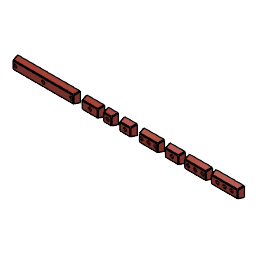
Keycaps Print (Autodesk Fusion 360 design; units mm, degrees)
part number: 2026-04-15-17-36-02-088
Autodesk Fusion 360 part; units mm, degrees
(part 1 of 2)
sketch "Sketch1" plane through (0, 0, 0) normal (0, 1, 0) x (1, 0, 0)
  line L0 (0, 0) -> (18, 0)
  line L1 (18, 0) -> (18, 18)
  line L2 (18, 18) -> (0, 18)
  line L3 (0, 18) -> (0, 0)
  dimension "d1" = 18
  dimension "d2" = 18
  constraint horizontal L0
  constraint vertical L1
  constraint horizontal L2
  constraint vertical L3
  constraint coincident L0.start L3.end
  measures "d1" distance of L0.start L0.end
  measures "d2" distance of L0.start L2.end
extrude "Extrude1" add sketch "Sketch1" along normal blind 10 makes body 1
sketch "Sketch2" plane through (0, 0, 0) normal (0, 0, 1) x (1, 0, 0)
  line L0 (0, 0) -> (18, 0)
  line L1 (18, 0) -> (18, 10)
  line L2 (18, 10) -> (0, 10)
  line L3 (0, 10) -> (0, 0)
  line L4 (0, 10) -> (2, 10)
  line L5 (2, 10) -> (0, 0)
  line L6 (0, 0) -> (0, 10)
  line L7 (18, 10) -> (16, 10)
  line L8 (16, 10) -> (18, 0)
  line L9 (18, 0) -> (18, 10)
  constraint coincident L2.end L3.start
  constraint coincident L2 L4.end
  constraint coincident L0.start L3.end
  constraint coincident L1.end L2.start
  constraint coincident L2 L7.end
  constraint coincident L0.end L1.start
sketch "Sketch3" plane through (18, 0, 0) normal (1, 0, 0) x (0, 0, -1)
  line L0 (0, 0) -> (18, 0)
  line L1 (18, 0) -> (18, 10)
  line L2 (18, 10) -> (0, 10)
  line L3 (0, 10) -> (0, 0)
  line L4 (0, 10) -> (2, 10)
  line L5 (2, 10) -> (0, 0)
  line L6 (0, 0) -> (0, 10)
  line L7 (18, 10) -> (16, 10)
  line L8 (16, 10) -> (18, 0)
  line L9 (18, 0) -> (18, 10)
  constraint coincident L2.end L3.start
  constraint coincident L2 L4.end
  constraint coincident L0.start L3.end
  constraint coincident L1.end L2.start
  constraint coincident L2 L7.end
  constraint coincident L0.end L1.start
extrude "Extrude2" cut sketch "Sketch3" against normal blind 39 contours L2 L3 L4 L5 L6 | L1 L2 L7 L8 L9 bodies 1
extrude "Extrude3" cut sketch "Sketch2" against normal blind 27 contours L2 L3 L4 L5 L6 | L1 L2 L7 L8 L9 bodies 1
shell "Shell2" thickness 1 removed faces 1 at (6, 0, -12) on bodies 1
sketch "Sketch4" plane through (0, 9, 0) normal (0, -1, 0) x (1, 0, 0)
  line L0 (15.1802, -15.1802) -> (15.1802, -2.8198)
  line L1 (15.1802, -2.8198) -> (2.8198, -2.8198)
  line L2 (2.8198, -2.8198) -> (2.8198, -15.1802)
  line L3 (2.8198, -15.1802) -> (15.1802, -15.1802)
  line L4 (8.45, -11) -> (9.55, -11)
  line L5 (9.55, -11) -> (9.55, -7)
  line L6 (9.55, -7) -> (8.45, -7)
  line L7 (8.45, -7) -> (8.45, -11)
  line L8 (7, -8.375) -> (11, -8.375)
  line L9 (11, -8.375) -> (11, -9.625)
  line L10 (11, -9.625) -> (7, -9.625)
  line L11 (7, -9.625) -> (7, -8.375)
  line L12 (10.55, -6) -> (7.45, -6)
  line L13 (7.45, -6) -> (7.45, -12)
  line L14 (7.45, -12) -> (10.55, -12)
  line L15 (10.55, -12) -> (10.55, -6)
  line L16 (12, -10.625) -> (6, -10.625)
  line L17 (6, -10.625) -> (6, -7.375)
  line L18 (6, -7.375) -> (12, -7.375)
  line L19 (12, -7.375) -> (12, -10.625)
  dimension "d21" = 3.1
  dimension "d22" = 6
  dimension "d25" = 6
  dimension "d26" = 3.25
  constraint horizontal L4
  constraint vertical L5
  constraint horizontal L6
  constraint vertical L7
  constraint horizontal L8
  constraint vertical L9
  constraint horizontal L10
  constraint vertical L11
  constraint horizontal L12
  constraint vertical L13
  constraint horizontal L14
  constraint vertical L15
  constraint horizontal L16
  constraint vertical L17
  constraint horizontal L18
  constraint vertical L19
  measures "d21" distance of L12.start L12.end
  measures "d22" distance of L12.start L14.end
  measures "d25" distance of L16.start L16.end
  measures "d26" distance of L16.start L18.end
extrude "Extrude4" add sketch "Sketch4" along normal blind 9 contours L4 L5 L7 L13 L14 L15 L16 | L7 L10 L13 L16 | L5 L10 L15 L16 | L8 L10 L11 L13 L16 L17 L18 | L8 L9 L10 L15 L16 L18 L19 | L7 L8 L13 L18 | L5 L8 L15 L18 | L5 L6 L7 L12 L13 L15 L18 bodies 1
fillet "Fillet1" radius 1 8 edges at (16, 10, -9) (9, 10, -16) (2, 10, -9) (9, 10, -2) (1, 5, -17) (1, 5, -1) (17, 5, -1) (17, 5, -17) on bodies 1
move_body "Move1" bodies 1 to x (1, 0, 0) y (0, 0, 1) z (0, -1, 0) at (-9, -1.3198, -24.8198)
move_body "Move2" bodies 1 to x (1, 0, 0) y (0, 1, 0) z (0, 0, 1) at (0, -7, 37)
sketch "Sketch5" plane through (0, 0, 0) normal (0, 0, 1) x (1, 0, 0)
  line L0 (25, 0) -> (133, 0)
  line L1 (133, 0) -> (133, 18)
  line L2 (133, 18) -> (25, 18)
  line L3 (25, 18) -> (25, 0)
  dimension "d31" = 108
  dimension "d32" = 18
  constraint horizontal L0
  constraint vertical L1
  constraint horizontal L2
  constraint vertical L3
  measures "d31" distance of L0.start L0.end
  measures "d32" distance of L0.start L2.end
extrude "Extrude5" add sketch "Sketch5" along normal blind 10 separate body makes body 2
sketch "Sketch6" plane through (0, 0, 0) normal (0, -1, 0) x (1, 0, 0)
  line L0 (25, 0) -> (133, 0)
  line L1 (133, 0) -> (133, 10)
  line L2 (133, 10) -> (25, 10)
  line L3 (25, 10) -> (25, 0)
  line L4 (25, 10) -> (27, 10)
  line L5 (27, 10) -> (25, 0)
  line L6 (25, 0) -> (25, 10)
  line L7 (133, 10) -> (131, 10)
  line L8 (131, 10) -> (133, 0)
  line L9 (133, 0) -> (133, 10)
  constraint coincident L2.end L3.start
  constraint coincident L2 L4.end
  constraint coincident L0.start L3.end
  constraint coincident L1.end L2.start
  constraint coincident L2 L7.end
  constraint coincident L0.end L1.start
sketch "Sketch7" plane through (133, 0, 0) normal (1, 0, 0) x (0, 0, -1)
  line L0 (0, 0) -> (0, 18)
  line L1 (0, 18) -> (-10, 18)
  line L2 (-10, 18) -> (-10, 0)
  line L3 (-10, 0) -> (0, 0)
  line L4 (-10, 0) -> (-10, 2)
  line L5 (-10, 2) -> (0, 0)
  line L6 (0, 0) -> (-10, 0)
  line L7 (-10, 18) -> (-10, 16)
  line L8 (-10, 16) -> (0, 18)
  line L9 (0, 18) -> (-10, 18)
  constraint coincident L2.end L3.start
  constraint coincident L2 L4.end
  constraint coincident L0.start L3.end
  constraint coincident L1.end L2.start
  constraint coincident L2 L7.end
  constraint coincident L0.end L1.start
extrude "Extrude6" cut sketch "Sketch7" against normal blind 116 contours L2 L3 L4 L5 L6 | L1 L2 L7 L8 L9 bodies 2
extrude "Extrude7" cut sketch "Sketch6" against normal blind 20 contours L2 L3 L4 L5 L6 | L1 L2 L7 L8 L9 bodies 2
shell "Shell3" thickness 1 removed faces 1 at (61, 12, 0) on bodies 2
sketch "Sketch8" plane through (0, 0, 9) normal (0, 0, -1) x (-1, 0, 0)
  line L0 (-27.8198, 2.8198) -> (-27.8198, 15.1802)
  line L1 (-27.8198, 15.1802) -> (-130.1802, 15.1802)
  line L2 (-130.1802, 15.1802) -> (-130.1802, 2.8198)
  line L3 (-130.1802, 2.8198) -> (-27.8198, 2.8198)
  line L4 (-79.55, 7) -> (-78.45, 7)
  line L5 (-78.45, 7) -> (-78.45, 11)
  line L6 (-78.45, 11) -> (-79.55, 11)
  line L7 (-79.55, 11) -> (-79.55, 7)
  line L8 (-77, 8.375) -> (-81, 8.375)
  line L9 (-81, 8.375) -> (-81, 9.625)
  line L10 (-81, 9.625) -> (-77, 9.625)
  line L11 (-77, 9.625) -> (-77, 8.375)
  line L12 (-80.55, 6) -> (-77.45, 6)
  line L13 (-77.45, 6) -> (-77.45, 12)
  line L14 (-77.45, 12) -> (-80.55, 12)
  line L15 (-80.55, 12) -> (-80.55, 6)
  line L16 (-82, 7.375) -> (-76, 7.375)
  line L17 (-76, 7.375) -> (-76, 10.625)
  line L18 (-76, 10.625) -> (-82, 10.625)
  line L19 (-82, 10.625) -> (-82, 7.375)
  line L20 (-123.788, 10.625) -> (-129.788, 10.625)
  line L21 (-129.788, 10.625) -> (-129.788, 7.375)
  line L22 (-129.788, 7.375) -> (-123.788, 7.375)
  line L23 (-123.788, 7.375) -> (-123.788, 10.625)
  line L24 (-128.788, 9.625) -> (-124.788, 9.625)
  line L25 (-124.788, 9.625) -> (-124.788, 8.375)
  line L26 (-128.788, 8.375) -> (-128.788, 9.625)
  line L27 (-124.788, 8.375) -> (-128.788, 8.375)
  line L28 (-127.338, 11) -> (-127.338, 7)
  line L29 (-127.338, 7) -> (-126.238, 7)
  line L30 (-126.238, 11) -> (-127.338, 11)
  line L31 (-126.238, 7) -> (-126.238, 11)
  line L32 (-128.338, 12) -> (-128.338, 6)
  line L33 (-128.338, 6) -> (-125.238, 6)
  line L34 (-125.238, 12) -> (-128.338, 12)
  line L35 (-125.238, 6) -> (-125.238, 12)
  line L36 (-76, 10.625) -> (-82, 10.625)
  line L37 (-82, 10.625) -> (-82, 7.375)
  line L38 (-82, 7.375) -> (-76, 7.375)
  line L39 (-76, 7.375) -> (-76, 10.625)
  line L40 (-81, 9.625) -> (-77, 9.625)
  line L41 (-77, 9.625) -> (-77, 8.375)
  line L42 (-81, 8.375) -> (-81, 9.625)
  line L43 (-77, 8.375) -> (-81, 8.375)
  line L44 (-79.55, 11) -> (-79.55, 7)
  line L45 (-79.55, 7) -> (-78.45, 7)
  line L46 (-78.45, 11) -> (-79.55, 11)
  line L47 (-78.45, 7) -> (-78.45, 11)
  line L48 (-80.55, 12) -> (-80.55, 6)
  line L49 (-80.55, 6) -> (-77.45, 6)
  line L50 (-77.45, 12) -> (-80.55, 12)
  line L51 (-77.45, 6) -> (-77.45, 12)
  line L52 (-28.212, 10.625) -> (-34.212, 10.625)
  line L53 (-34.212, 10.625) -> (-34.212, 7.375)
  line L54 (-34.212, 7.375) -> (-28.212, 7.375)
  line L55 (-28.212, 7.375) -> (-28.212, 10.625)
  line L56 (-33.212, 9.625) -> (-29.212, 9.625)
  line L57 (-29.212, 9.625) -> (-29.212, 8.375)
  line L58 (-33.212, 8.375) -> (-33.212, 9.625)
  line L59 (-29.212, 8.375) -> (-33.212, 8.375)
  line L60 (-31.762, 11) -> (-31.762, 7)
  line L61 (-31.762, 7) -> (-30.662, 7)
  line L62 (-30.662, 11) -> (-31.762, 11)
  line L63 (-30.662, 7) -> (-30.662, 11)
  line L64 (-32.762, 12) -> (-32.762, 6)
  line L65 (-32.762, 6) -> (-29.662, 6)
  line L66 (-29.662, 12) -> (-32.762, 12)
  line L67 (-29.662, 6) -> (-29.662, 12)
  dimension "d46" = 3.1
  dimension "d47" = 6
  dimension "d50" = 6
  dimension "d51" = 3.25
  dimension "d56" = 3.1
  dimension "d57" = 6
  dimension "d58" = 6
  dimension "d59" = 3.25
  dimension "d60" = 3.1
  dimension "d61" = 6
  dimension "d62" = 6
  dimension "d63" = 3.25
  dimension "d64" = 3.1
  dimension "d65" = 6
  dimension "d66" = 6
  dimension "d67" = 3.25
  constraint horizontal L4
  constraint vertical L5
  constraint horizontal L6
  constraint vertical L7
  constraint horizontal L8
  constraint vertical L9
  constraint horizontal L10
  constraint vertical L11
  constraint horizontal L12
  constraint vertical L13
  constraint horizontal L14
  constraint vertical L15
  constraint horizontal L16
  constraint vertical L17
  constraint horizontal L18
  constraint vertical L19
  constraint horizontal L29
  constraint vertical L31
  constraint horizontal L30
  constraint vertical L28
  constraint horizontal L27
  constraint vertical L26
  constraint horizontal L24
  constraint vertical L25
  constraint horizontal L33
  constraint vertical L35
  constraint horizontal L34
  constraint vertical L32
  constraint horizontal L22
  constraint vertical L23
  constraint horizontal L20
  constraint vertical L21
  constraint horizontal L45
  constraint vertical L47
  constraint horizontal L46
  constraint vertical L44
  constraint horizontal L43
  constraint vertical L42
  constraint horizontal L40
  constraint vertical L41
  constraint horizontal L49
  constraint vertical L51
  constraint horizontal L50
  constraint vertical L48
  constraint horizontal L38
  constraint vertical L39
  constraint horizontal L36
  constraint vertical L37
  constraint horizontal L61
  constraint vertical L63
  constraint horizontal L62
  constraint vertical L60
  constraint horizontal L59
  constraint vertical L58
  constraint horizontal L56
  constraint vertical L57
  constraint horizontal L65
  constraint vertical L67
  constraint horizontal L66
  constraint vertical L64
  constraint horizontal L54
  constraint vertical L55
  constraint horizontal L52
  constraint vertical L53
  measures "d46" distance of L12.start L12.end
  measures "d47" distance of L12.start L14.end
  measures "d50" distance of L16.start L16.end
  measures "d51" distance of L16.start L18.end
  measures "d56" distance of L33.end L32.end
  measures "d57" distance of L32.start L32.end
  measures "d58" distance of L22.end L21.end
  measures "d59" distance of L20.end L21.end
  measures "d60" distance of L12.end L12.start
  measures "d61" distance of L14.end L12.start
  measures "d62" distance of L16.end L16.start
  measures "d63" distance of L18.end L16.start
  measures "d64" distance of L65.end L64.end
  measures "d65" distance of L64.start L64.end
  measures "d66" distance of L54.end L53.end
  measures "d67" distance of L52.end L53.end
extrude "Extrude8" add sketch "Sketch8" along normal blind 9 contours L4 L5 L7 L12 L13 L15 L16 L38 L44 L45 L47 L48 L49 L51 | L7 L8 L15 L16 L38 L43 L44 L48 | L5 L8 L13 L16 L38 L43 L47 L51 | L8 L9 L10 L15 L16 L18 L19 L36 L37 L38 L40 L42 L43 L48 | L8 L10 L11 L13 L16 L17 L18 L36 L38 L39 L40 L41 L43 L51 | L7 L10 L15 L18 L36 L40 L44 L48 | L5 L10 L13 L18 L36 L40 L47 L51 | L5 L6 L7 L13 L14 L15 L18 L36 L44 L46 L47 L48 L50 L51 bodies 2
fillet "Fillet2" radius 1 8 edges at (79, 16, 10) (27, 9, 10) (26, 17, 5) (26, 1, 5) (79, 2, 10) (132, 17, 5) (131, 9, 10) (132, 1, 5) on bodies 2
extrude "Extrude9" add sketch "Sketch8" along normal blind 9 contours L20 L22 L23 L24 L25 L27 L35 | L20 L24 L31 L35 | L20 L28 L30 L31 L32 L34 L35 | L22 L28 L29 L31 L32 L33 L35 | L22 L27 L31 L35 | L20 L24 L28 L32 | L20 L21 L22 L24 L26 L27 L32 | L22 L27 L28 L32 | L52 L54 L55 L56 L57 L59 L67 | L52 L56 L63 L67 | L52 L60 L62 L63 L64 L66 L67 | L54 L60 L61 L63 L64 L65 L67 | L54 L59 L63 L67 | L52 L56 L60 L64 | L52 L53 L54 L56 L58 L59 L64 | L54 L59 L60 L64 bodies 2
move_body "Move3" bodies 2 to x (1, 0, 0) y (0, 1, 0) z (0, 0, 1) at (-78.996, -8.312, 15)
move_body "Move4" bodies 2 to x (1, 0, 0) y (0, 1, 0) z (0, 0, 1) at (0, 0, -2.8)
sketch "Sketch9" plane through (0, 0, 0) normal (0, 0, 1) x (1, 0, 0)
  line L0 (-75, 0) -> (-97.5, 0)
  line L1 (-97.5, 0) -> (-97.5, -18)
  line L2 (-97.5, -18) -> (-75, -18)
  line L3 (-75, -18) -> (-75, 0)
  dimension "d70" = 22.5
  dimension "d71" = 18
  constraint horizontal L0
  constraint vertical L1
  constraint horizontal L2
  constraint vertical L3
  measures "d70" distance of L0.start L0.end
  measures "d71" distance of L0.start L2.end
extrude "Extrude10" add sketch "Sketch9" along normal blind 10 separate body makes body 3
sketch "Sketch10" plane through (0, 0, 0) normal (0, 1, 0) x (-1, 0, 0)
  line L0 (75, 0) -> (97.5, 0)
  line L1 (97.5, 0) -> (97.5, 10)
  line L2 (97.5, 10) -> (75, 10)
  line L3 (75, 10) -> (75, 0)
  line L4 (75, 10) -> (77, 10)
  line L5 (77, 10) -> (75, 0)
  line L6 (75, 0) -> (75, 10)
  line L7 (97.5, 10) -> (95.5, 10)
  line L8 (95.5, 10) -> (97.5, 0)
  line L9 (97.5, 0) -> (97.5, 10)
  dimension "d74" = 2
  constraint coincident L2.end L3.start
  constraint coincident L2 L4.end
  constraint coincident L0.start L3.end
  constraint coincident L1.end L2.start
  constraint perpendicular L1 L7
  constraint coincident L0.end L1.start
  measures "d74" distance of L1.end L7.end
sketch "Sketch11" plane through (-97.5, 0, 0) normal (-1, 0, 0) x (0, 0, 1)
  line L0 (0, 0) -> (0, -18)
  line L1 (0, -18) -> (10, -18)
  line L2 (10, -18) -> (10, 0)
  line L3 (10, 0) -> (0, 0)
  line L4 (10, 0) -> (10, -2)
  line L5 (10, -2) -> (0, 0)
  line L6 (0, 0) -> (10, 0)
  line L7 (10, -18) -> (10, -16)
  line L8 (10, -16) -> (0, -18)
  line L9 (0, -18) -> (10, -18)
  constraint coincident L2.end L3.start
  constraint coincident L2 L4.end
  constraint coincident L0.start L3.end
  constraint coincident L1.end L2.start
  constraint coincident L2 L7.end
  constraint coincident L0.end L1.start
extrude "Extrude11" cut sketch "Sketch11" against normal blind 27 contours L2 L3 L4 L5 L6 | L1 L2 L7 L8 L9 bodies 3
extrude "Extrude12" cut sketch "Sketch10" against normal blind 26 contours L2 L3 L4 L5 L6 | L1 L2 L7 L8 L9 bodies 3
shell "Shell4" thickness 1 removed faces 1 at (-90, -6, 0) on bodies 3
sketch "Sketch12" plane through (0, 0, 9) normal (0, 0, -1) x (-1, 0, 0)
  line L0 (94.6802, -15.1802) -> (94.6802, -2.8198)
  line L1 (94.6802, -2.8198) -> (77.8198, -2.8198)
  line L2 (77.8198, -2.8198) -> (77.8198, -15.1802)
  line L3 (77.8198, -15.1802) -> (94.6802, -15.1802)
  line L4 (85.7, -11) -> (86.8, -11)
  line L5 (86.8, -11) -> (86.8, -7)
  line L6 (86.8, -7) -> (85.7, -7)
  line L7 (85.7, -7) -> (85.7, -11)
  line L8 (84.25, -8.375) -> (88.25, -8.375)
  line L9 (88.25, -8.375) -> (88.25, -9.625)
  line L10 (88.25, -9.625) -> (84.25, -9.625)
  line L11 (84.25, -9.625) -> (84.25, -8.375)
  line L12 (87.8, -6) -> (84.7, -6)
  line L13 (84.7, -6) -> (84.7, -12)
  line L14 (84.7, -12) -> (87.8, -12)
  line L15 (87.8, -12) -> (87.8, -6)
  line L16 (89.25, -10.625) -> (83.25, -10.625)
  line L17 (83.25, -10.625) -> (83.25, -7.375)
  line L18 (83.25, -7.375) -> (89.25, -7.375)
  line L19 (89.25, -7.375) -> (89.25, -10.625)
  dimension "d90" = 3.1
  dimension "d91" = 6
  dimension "d94" = 6
  dimension "d95" = 3.25
  constraint horizontal L4
  constraint vertical L5
  constraint horizontal L6
  constraint vertical L7
  constraint horizontal L8
  constraint vertical L9
  constraint horizontal L10
  constraint vertical L11
  constraint horizontal L12
  constraint vertical L13
  constraint horizontal L14
  constraint vertical L15
  constraint horizontal L16
  constraint vertical L17
  constraint horizontal L18
  constraint vertical L19
  measures "d90" distance of L12.start L12.end
  measures "d91" distance of L12.start L14.end
  measures "d94" distance of L16.start L16.end
  measures "d95" distance of L16.start L18.end
extrude "Extrude13" add sketch "Sketch12" along normal blind 9 contours L4 L5 L7 L13 L14 L15 L16 | L7 L10 L13 L16 | L5 L10 L15 L16 | L8 L10 L11 L13 L16 L17 L18 | L8 L9 L10 L15 L16 L18 L19 | L7 L8 L13 L18 | L5 L8 L15 L18 | L5 L6 L7 L12 L13 L15 L18 bodies 3
fillet "Fillet3" radius 1 8 edges at (-86.25, -16, 10) (-76, -17, 5) (-77, -9, 10) (-76, -1, 5) (-86.25, -2, 10) (-96.5, -17, 5) (-95.5, -9, 10) (-96.5, -1, 5) on bodies 3
move_body "Move5" bodies 3 to x (1, 0, 0) y (0, 1, 0) z (0, 0, 1) at (86.2551, 9.6865, 12)
move_body "Move6" bodies 3 to x (1, 0, 0) y (0, 1, 0) z (0, 0, 1) at (0, 0, 0.2)
sketch "Sketch13" plane through (0, 0, 0) normal (0, 0, 1) x (1, 0, 0)
  line L0 (20, 0) -> (56, 0)
  line L1 (56, 0) -> (56, 18)
  line L2 (56, 18) -> (20, 18)
  line L3 (20, 18) -> (20, 0)
  dimension "d100" = 36
  dimension "d101" = 18
  constraint horizontal L0
  constraint vertical L1
  constraint horizontal L2
  constraint vertical L3
  measures "d100" distance of L0.start L0.end
  measures "d101" distance of L0.start L2.end
extrude "Extrude14" add sketch "Sketch13" along normal blind 10 separate body makes body 4
sketch "Sketch14" plane through (0, 0, 0) normal (0, -1, 0) x (1, 0, 0)
  line L0 (20, 0) -> (56, 0)
  line L1 (56, 0) -> (56, 10)
  line L2 (56, 10) -> (20, 10)
  line L3 (20, 10) -> (20, 0)
  line L4 (20, 10) -> (22, 10)
  line L5 (22, 10) -> (20, 0)
  line L6 (20, 0) -> (20, 10)
  line L7 (56, 10) -> (54, 10)
  line L8 (54, 10) -> (56, 0)
  line L9 (56, 0) -> (56, 10)
  constraint coincident L2.end L3.start
  constraint coincident L2 L4.end
  constraint coincident L0.start L3.end
  constraint coincident L1.end L2.start
  constraint coincident L2 L7.end
  constraint coincident L0.end L1.start
sketch "Sketch15" plane through (56, 0, 0) normal (1, 0, 0) x (0, 0, -1)
  line L0 (0, 0) -> (0, 18)
  line L1 (0, 18) -> (-10, 18)
  line L2 (-10, 18) -> (-10, 0)
  line L3 (-10, 0) -> (0, 0)
  line L4 (-10, 0) -> (-10, 2)
  line L5 (-10, 2) -> (0, 0)
  line L6 (0, 0) -> (-10, 0)
  line L7 (-10, 18) -> (-10, 16)
  line L8 (-10, 16) -> (0, 18)
  line L9 (0, 18) -> (-10, 18)
  constraint coincident L2.end L3.start
  constraint coincident L2 L4.end
  constraint coincident L0.start L3.end
  constraint coincident L1.end L2.start
  constraint coincident L2 L7.end
  constraint coincident L0.end L1.start
extrude "Extrude15" cut sketch "Sketch15" against normal blind 41 contours L2 L3 L4 L5 L6 | L1 L2 L7 L8 L9 bodies 4
extrude "Extrude16" cut sketch "Sketch14" against normal blind 32 contours L2 L3 L4 L5 L6 | L1 L2 L7 L8 L9 bodies 4
shell "Shell5" thickness 1 removed faces 1 at (32, 12, 0) on bodies 4
sketch "Sketch16" plane through (0, 0, 9) normal (0, 0, -1) x (-1, 0, 0)
  line L0 (-22.8198, 2.8198) -> (-22.8198, 15.1802)
  line L1 (-22.8198, 15.1802) -> (-53.1802, 15.1802)
  line L2 (-53.1802, 15.1802) -> (-53.1802, 2.8198)
  line L3 (-53.1802, 2.8198) -> (-22.8198, 2.8198)
  line L4 (-38.55, 7) -> (-37.45, 7)
  line L5 (-37.45, 7) -> (-37.45, 11)
  line L6 (-37.45, 11) -> (-38.55, 11)
  line L7 (-38.55, 11) -> (-38.55, 7)
  line L8 (-38, 9) -> (-40, 9)
  line L9 (-40, 9) -> (-40, 9.625)
  line L10 (-40, 9.625) -> (-36, 9.625)
  line L11 (-36, 9.625) -> (-36, 8.375)
  line L12 (-36, 8.375) -> (-40, 8.375)
  line L13 (-40, 8.375) -> (-40, 9.625)
  line L14 (-39.55, 6) -> (-36.45, 6)
  line L15 (-36.45, 6) -> (-36.45, 12)
  line L16 (-36.45, 12) -> (-39.55, 12)
  line L17 (-39.55, 12) -> (-39.55, 6)
  line L18 (-35, 7.375) -> (-41, 7.375)
  line L19 (-41, 7.375) -> (-41, 10.625)
  line L20 (-41, 10.625) -> (-35, 10.625)
  line L21 (-35, 10.625) -> (-35, 7.375)
  line L22 (-22.922, 10.625) -> (-22.922, 7.375)
  line L23 (-22.922, 7.375) -> (-28.922, 7.375)
  line L24 (-28.922, 7.375) -> (-28.922, 10.625)
  line L25 (-28.922, 10.625) -> (-22.922, 10.625)
  line L26 (-24.372, 6) -> (-24.372, 12)
  line L27 (-24.372, 12) -> (-27.472, 12)
  line L28 (-27.472, 6) -> (-24.372, 6)
  line L29 (-27.472, 12) -> (-27.472, 6)
  line L30 (-23.922, 9.625) -> (-23.922, 8.375)
  line L31 (-23.922, 8.375) -> (-27.922, 8.375)
  line L32 (-27.922, 8.375) -> (-27.922, 9.625)
  line L33 (-27.922, 9.625) -> (-23.922, 9.625)
  line L34 (-25.372, 7) -> (-25.372, 11)
  line L35 (-25.372, 11) -> (-26.472, 11)
  line L36 (-26.472, 7) -> (-25.372, 7)
  line L37 (-26.472, 11) -> (-26.472, 7)
  line L38 (-47.078, 10.625) -> (-47.078, 7.375)
  line L39 (-47.078, 7.375) -> (-53.078, 7.375)
  line L40 (-53.078, 7.375) -> (-53.078, 10.625)
  line L41 (-53.078, 10.625) -> (-47.078, 10.625)
  line L42 (-48.528, 6) -> (-48.528, 12)
  line L43 (-48.528, 12) -> (-51.628, 12)
  line L44 (-51.628, 6) -> (-48.528, 6)
  line L45 (-51.628, 12) -> (-51.628, 6)
  line L46 (-48.078, 9.625) -> (-48.078, 8.375)
  line L47 (-48.078, 8.375) -> (-52.078, 8.375)
  line L48 (-52.078, 8.375) -> (-52.078, 9.625)
  line L49 (-52.078, 9.625) -> (-48.078, 9.625)
  line L50 (-49.528, 7) -> (-49.528, 11)
  line L51 (-49.528, 11) -> (-50.628, 11)
  line L52 (-50.628, 7) -> (-49.528, 7)
  line L53 (-50.628, 11) -> (-50.628, 7)
  dimension "d112" = 1.1
  dimension "d113" = 4
  dimension "d115" = 2
  dimension "d116" = 0.625
  dimension "d117" = 4
  dimension "d118" = 1.25
  dimension "d121" = 3.1
  dimension "d122" = 6
  dimension "d125" = 6
  dimension "d126" = 3.25
  dimension "d131" = 1.1
  dimension "d132" = 4
  dimension "d133" = 4
  dimension "d134" = 1.25
  dimension "d135" = 3.1
  dimension "d136" = 6
  dimension "d137" = 6
  dimension "d138" = 3.25
  dimension "d139" = 1.1
  dimension "d140" = 4
  dimension "d141" = 4
  dimension "d142" = 1.25
  dimension "d143" = 3.1
  dimension "d144" = 6
  dimension "d145" = 6
  dimension "d146" = 3.25
  constraint horizontal L4
  constraint vertical L5
  constraint horizontal L6
  constraint vertical L7
  constraint perpendicular L5 L8
  constraint perpendicular L8 L9
  constraint horizontal L10
  constraint vertical L11
  constraint horizontal L12
  constraint vertical L13
  constraint horizontal L14
  constraint vertical L15
  constraint horizontal L16
  constraint vertical L17
  constraint horizontal L18
  constraint vertical L19
  constraint horizontal L20
  constraint vertical L21
  constraint horizontal L36
  constraint vertical L34
  constraint horizontal L35
  constraint vertical L37
  constraint horizontal L33
  constraint vertical L30
  constraint horizontal L31
  constraint vertical L32
  constraint horizontal L28
  constraint vertical L26
  constraint horizontal L27
  constraint vertical L29
  constraint horizontal L23
  constraint vertical L24
  constraint horizontal L25
  constraint vertical L22
  constraint horizontal L52
  constraint vertical L50
  constraint horizontal L51
  constraint vertical L53
  constraint horizontal L49
  constraint vertical L46
  constraint horizontal L47
  constraint vertical L48
  constraint horizontal L44
  constraint vertical L42
  constraint horizontal L43
  constraint vertical L45
  constraint horizontal L39
  constraint vertical L40
  constraint horizontal L41
  constraint vertical L38
  measures "d112" distance of L4.start L4.end
  measures "d113" distance of L4.start L6.end
  measures "d115" distance of L8.start L8.end
  measures "d116" distance of L8.end L9.end
  measures "d117" distance of L9.end L10.end
  measures "d118" distance of L9.end L12.end
  measures "d121" distance of L14.start L14.end
  measures "d122" distance of L14.start L16.end
  measures "d125" distance of L18.start L18.end
  measures "d126" distance of L18.start L20.end
  measures "d131" distance of L36.start L34.start
  measures "d132" distance of L36.start L35.end
  measures "d133" distance of L32.end L30.start
  measures "d134" distance of L32.end L31.end
  measures "d135" distance of L28.start L26.start
  measures "d136" distance of L27.end L28.start
  measures "d137" distance of L23.end L22.end
  measures "d138" distance of L22.end L22.start
  measures "d139" distance of L52.start L50.start
  measures "d140" distance of L52.start L51.end
  measures "d141" distance of L48.end L46.start
  measures "d142" distance of L48.end L47.end
  measures "d143" distance of L44.start L42.start
  measures "d144" distance of L43.end L44.start
  measures "d145" distance of L39.end L38.end
  measures "d146" distance of L38.end L38.start
extrude "Extrude17" add sketch "Sketch16" along normal blind 9 contours L4 L5 L7 L14 L15 L17 L18 | L7 L12 L17 L18 | L5 L12 L15 L18 | L9 L10 L12 L13 L17 L18 L19 L20 | L10 L11 L12 L15 L18 L20 L21 | L5 L10 L15 L20 | L7 L10 L17 L20 | L5 L6 L7 L15 L16 L17 L20 bodies 4
extrude "Extrude18" add sketch "Sketch16" along normal blind 9 contours L22 L23 L25 L26 L30 L31 L33 | L25 L26 L33 L34 | L25 L26 L27 L29 L34 L35 L37 | L23 L26 L28 L29 L34 L36 L37 | L23 L26 L31 L34 | L25 L29 L33 L37 | L23 L29 L31 L37 | L23 L24 L25 L29 L31 L32 L33 | L38 L39 L41 L42 L46 L47 L49 | L41 L42 L49 L50 | L41 L42 L43 L45 L50 L51 L53 | L39 L42 L44 L45 L50 L52 L53 | L39 L42 L47 L50 | L41 L45 L49 L53 | L39 L45 L47 L53 | L39 L40 L41 L45 L47 L48 L49 bodies 4
fillet "Fillet5" radius 1 8 edges at (38, 16, 10) (22, 9, 10) (21, 17, 5) (21, 1, 5) (38, 2, 10) (55, 17, 5) (54, 9, 10) (55, 1, 5) on bodies 4
move_body "Move7" bodies 4 to x (1, 0, 0) y (0, 1, 0) z (0, 0, 1) at (-37.9759, -8.2892, 12)
move_body "Move8" bodies 4 to x (1, 0, 0) y (0, 1, 0) z (0, 0, 1) at (-0.0354, -0.0473, 0)
move_body "Move9" bodies 4 to x (1, 0, 0) y (0, 1, 0) z (0, 0, 1) at (0, 0, 0.2)
sketch "Sketch17" plane through (0, 0, 0) normal (0, 0, 1) x (1, 0, 0)
  line L0 (-25, 0) -> (-52, 0)
  line L1 (-52, 0) -> (-52, -18)
  line L2 (-52, -18) -> (-25, -18)
  line L3 (-25, -18) -> (-25, 0)
  dimension "d150" = 27
  dimension "d151" = 18
  constraint horizontal L0
  constraint vertical L1
  constraint horizontal L2
  constraint vertical L3
  measures "d150" distance of L0.start L0.end
  measures "d151" distance of L0.start L2.end
extrude "Extrude19" add sketch "Sketch17" along normal blind 10 separate body makes body 5
sketch "Sketch18" plane through (0, 0, 0) normal (0, 1, 0) x (-1, 0, 0)
  line L0 (25, 0) -> (52, 0)
  line L1 (52, 0) -> (52, 10)
  line L2 (52, 10) -> (25, 10)
  line L3 (25, 10) -> (25, 0)
  line L4 (25, 10) -> (27, 10)
  line L5 (27, 10) -> (25, 0)
  line L6 (25, 0) -> (25, 10)
  line L7 (52, 10) -> (50, 10)
  line L8 (50, 10) -> (52, 0)
  line L9 (52, 0) -> (52, 10)
  constraint coincident L2.end L3.start
  constraint coincident L2 L4.end
  constraint coincident L0.start L3.end
  constraint coincident L1.end L2.start
  constraint coincident L2 L7.end
  constraint coincident L0.end L1.start
sketch "Sketch19" plane through (-25, 0, 0) normal (1, 0, 0) x (0, 0, -1)
  line L0 (0, -18) -> (0, 0)
  line L1 (0, 0) -> (-10, 0)
  line L2 (-10, 0) -> (-10, -18)
  line L3 (-10, -18) -> (0, -18)
  line L4 (-10, -18) -> (-10, -16)
  line L5 (-10, -16) -> (0, -18)
  line L6 (0, -18) -> (-10, -18)
  line L7 (-10, 0) -> (-10, -2)
  line L8 (-10, -2) -> (0, 0)
  line L9 (-10, 0) -> (0, 0)
  constraint coincident L2.end L3.start
  constraint coincident L2 L4.end
  constraint coincident L0.start L3.end
  constraint coincident L1.end L2.start
  constraint coincident L2 L7.end
  constraint coincident L0.end L1.start
extrude "Extrude21" cut sketch "Sketch19" against normal blind 33 contours L2 L3 L4 L5 L6 | L1 L2 L7 L8 L9 bodies 5
extrude "Extrude20" cut sketch "Sketch18" against normal blind 27 contours L2 L3 L4 L5 L6 | L1 L2 L7 L8 L9 bodies 5
shell "Shell6" thickness 1 removed faces 1 at (-43, -6, 0) on bodies 5
sketch "Sketch20" plane through (0, 0, 9) normal (0, 0, -1) x (-1, 0, 0)
  line L0 (49.1802, -15.1802) -> (49.1802, -2.8198)
  line L1 (49.1802, -2.8198) -> (27.8198, -2.8198)
  line L2 (27.8198, -2.8198) -> (27.8198, -15.1802)
  line L3 (27.8198, -15.1802) -> (49.1802, -15.1802)
  line L4 (37.95, -11) -> (39.05, -11)
  line L5 (39.05, -11) -> (39.05, -7)
  line L6 (39.05, -7) -> (37.95, -7)
  line L7 (37.95, -7) -> (37.95, -11)
  line L8 (40.5, -9.625) -> (36.5, -9.625)
  line L9 (36.5, -9.625) -> (36.5, -8.375)
  line L10 (36.5, -8.375) -> (40.5, -8.375)
  line L11 (40.5, -8.375) -> (40.5, -9.625)
  line L12 (36.95, -12) -> (40.05, -12)
  line L13 (40.05, -12) -> (40.05, -6)
  line L14 (40.05, -6) -> (36.95, -6)
  line L15 (36.95, -6) -> (36.95, -12)
  line L16 (41.5, -10.625) -> (35.5, -10.625)
  line L17 (35.5, -10.625) -> (35.5, -7.375)
  line L18 (35.5, -7.375) -> (41.5, -7.375)
  line L19 (41.5, -7.375) -> (41.5, -10.625)
  dimension "d165" = 3.1
  dimension "d166" = 6
  dimension "d168" = 6
  dimension "d169" = 3.25
  constraint horizontal L4
  constraint vertical L5
  constraint horizontal L6
  constraint vertical L7
  constraint horizontal L8
  constraint vertical L9
  constraint horizontal L10
  constraint vertical L11
  constraint horizontal L12
  constraint vertical L13
  constraint horizontal L14
  constraint vertical L15
  constraint horizontal L16
  constraint vertical L17
  constraint horizontal L18
  constraint vertical L19
  measures "d165" distance of L12.start L12.end
  measures "d166" distance of L12.start L14.end
  measures "d168" distance of L16.start L16.end
  measures "d169" distance of L16.start L18.end
extrude "Extrude22" add sketch "Sketch20" along normal blind 9 contours L4 L5 L7 L12 L13 L15 L16 | L7 L8 L15 L16 | L5 L8 L13 L16 | L8 L9 L10 L15 L16 L17 L18 | L8 L10 L11 L13 L16 L18 L19 | L7 L10 L15 L18 | L5 L10 L13 L18 | L5 L6 L7 L13 L14 L15 L18 bodies 5
fillet "Fillet6" radius 1 8 edges at (-38.5, -2, 10) (-51, -1, 5) (-50, -9, 10) (-51, -17, 5) (-38.5, -16, 10) (-27, -9, 10) (-26, -1, 5) (-26, -17, 5) on bodies 5
move_body "Move10" bodies 5 to x (1, 0, 0) y (0, 1, 0) z (0, 0, 1) at (38.4895, 9.6689, 12.1744)
sketch "Sketch21" plane through (0, 0, 0) normal (0, 0, 1) x (1, 0, 0)
  line L0 (25, 0) -> (65.5, 0)
  line L1 (65.5, 0) -> (65.5, 18)
  line L2 (65.5, 18) -> (25, 18)
  line L3 (25, 18) -> (25, 0)
  dimension "d174" = 40.5
  dimension "d175" = 18
  constraint horizontal L0
  constraint vertical L1
  constraint horizontal L2
  constraint vertical L3
  measures "d174" distance of L0.start L0.end
  measures "d175" distance of L0.start L2.end
extrude "Extrude23" add sketch "Sketch21" along normal blind 10 separate body makes body 6
sketch "Sketch22" plane through (0, 0, 0) normal (0, -1, 0) x (1, 0, 0)
  line L0 (25, 0) -> (65.5, 0)
  line L1 (65.5, 0) -> (65.5, 10)
  line L2 (65.5, 10) -> (25, 10)
  line L3 (25, 10) -> (25, 0)
  line L4 (65.5, 10) -> (63.5, 10)
  line L5 (63.5, 10) -> (65.5, 0)
  line L6 (65.5, 0) -> (65.5, 10)
  line L7 (25, 10) -> (27, 10)
  line L8 (27, 10) -> (25, 0)
  line L9 (25, 0) -> (25, 10)
  dimension "d178" = 2
  constraint coincident L1.end L2.start
  constraint coincident L2 L4.end
  constraint coincident L0.end L1.start
  constraint coincident L2.end L3.start
  constraint coincident L2 L7.end
  constraint coincident L0.start L3.end
  measures "d178" distance of L1.end L4.end
sketch "Sketch23" plane through (65.5, 0, 0) normal (1, 0, 0) x (0, 0, -1)
  line L0 (0, 0) -> (0, 18)
  line L1 (0, 18) -> (-10, 18)
  line L2 (-10, 18) -> (-10, 0)
  line L3 (-10, 0) -> (0, 0)
  line L4 (-10, 18) -> (-10, 16)
  line L5 (-10, 16) -> (0, 18)
  line L6 (0, 18) -> (-10, 18)
  line L7 (-10, 0) -> (-10, 2)
  line L8 (-10, 2) -> (0, 0)
  line L9 (0, 0) -> (-10, 0)
  constraint coincident L1.end L2.start
  constraint coincident L2 L4.end
  constraint coincident L0.end L1.start
  constraint coincident L2.end L3.start
  constraint coincident L2 L7.end
  constraint coincident L0.start L3.end
extrude "Extrude24" cut sketch "Sketch23" against normal blind 45 contours L2 L3 L7 L8 L9 | L1 L2 L4 L5 L6 bodies 6
extrude "Extrude25" cut sketch "Sketch22" against normal blind 22 contours L2 L3 L7 L8 L9 | L1 L2 L4 L5 L6 bodies 6
shell "Shell7" thickness 1 removed faces 1 at (38.5, 12, 0) on bodies 6
sketch "Sketch24" plane through (0, 0, 9) normal (0, 0, -1) x (-1, 0, 0)
  line L0 (-62.6802, 15.1802) -> (-62.6802, 2.8198)
  line L1 (-62.6802, 2.8198) -> (-27.8198, 2.8198)
  line L2 (-27.8198, 2.8198) -> (-27.8198, 15.1802)
  line L3 (-27.8198, 15.1802) -> (-62.6802, 15.1802)
  line L4 (-45.8, 7) -> (-44.7, 7)
  line L5 (-44.7, 7) -> (-44.7, 11)
  line L6 (-44.7, 11) -> (-45.8, 11)
  line L7 (-45.8, 11) -> (-45.8, 7)
  line L8 (-43.25, 8.375) -> (-47.25, 8.375)
  line L9 (-47.25, 8.375) -> (-47.25, 9.625)
  line L10 (-47.25, 9.625) -> (-43.25, 9.625)
  line L11 (-43.25, 9.625) -> (-43.25, 8.375)
  line L12 (-46.8, 6) -> (-43.7, 6)
  line L13 (-43.7, 6) -> (-43.7, 12)
  line L14 (-43.7, 12) -> (-46.8, 12)
  line L15 (-46.8, 12) -> (-46.8, 6)
  line L16 (-48.25, 10.625) -> (-42.25, 10.625)
  line L17 (-42.25, 10.625) -> (-42.25, 7.375)
  line L18 (-42.25, 7.375) -> (-48.25, 7.375)
  line L19 (-48.25, 7.375) -> (-48.25, 10.625)
  line L20 (-30.175, 10.625) -> (-30.175, 7.375)
  line L21 (-30.175, 7.375) -> (-36.175, 7.375)
  line L22 (-36.175, 7.375) -> (-36.175, 10.625)
  line L23 (-36.175, 10.625) -> (-30.175, 10.625)
  line L24 (-31.625, 12) -> (-34.725, 12)
  line L25 (-34.725, 12) -> (-34.725, 6)
  line L26 (-31.625, 6) -> (-31.625, 12)
  line L27 (-34.725, 6) -> (-31.625, 6)
  line L28 (-32.625, 11) -> (-33.725, 11)
  line L29 (-33.725, 11) -> (-33.725, 7)
  line L30 (-32.625, 7) -> (-32.625, 11)
  line L31 (-33.725, 7) -> (-32.625, 7)
  line L32 (-35.175, 9.625) -> (-31.175, 9.625)
  line L33 (-31.175, 9.625) -> (-31.175, 8.375)
  line L34 (-35.175, 8.375) -> (-35.175, 9.625)
  line L35 (-31.175, 8.375) -> (-35.175, 8.375)
  line L36 (-54.325, 10.625) -> (-54.325, 7.375)
  line L37 (-54.325, 7.375) -> (-60.325, 7.375)
  line L38 (-60.325, 7.375) -> (-60.325, 10.625)
  line L39 (-60.325, 10.625) -> (-54.325, 10.625)
  line L40 (-55.325, 8.375) -> (-59.325, 8.375)
  line L41 (-59.325, 8.375) -> (-59.325, 9.625)
  line L42 (-55.325, 9.625) -> (-55.325, 8.375)
  line L43 (-59.325, 9.625) -> (-55.325, 9.625)
  line L44 (-56.775, 7) -> (-56.775, 11)
  line L45 (-56.775, 11) -> (-57.875, 11)
  line L46 (-57.875, 7) -> (-56.775, 7)
  line L47 (-57.875, 11) -> (-57.875, 7)
  line L48 (-58.875, 6) -> (-55.775, 6)
  line L49 (-55.775, 6) -> (-55.775, 12)
  line L50 (-58.875, 12) -> (-58.875, 6)
  line L51 (-55.775, 12) -> (-58.875, 12)
  dimension "d194" = 3.1
  dimension "d195" = 6
  dimension "d198" = 6
  dimension "d199" = 3.25
  dimension "d200" = 3.1
  dimension "d201" = 6
  dimension "d202" = 6
  dimension "d203" = 3.25
  dimension "d204" = 3.1
  dimension "d205" = 6
  dimension "d206" = 6
  dimension "d207" = 3.25
  constraint horizontal L4
  constraint vertical L5
  constraint horizontal L6
  constraint vertical L7
  constraint horizontal L8
  constraint vertical L9
  constraint horizontal L10
  constraint vertical L11
  constraint horizontal L12
  constraint vertical L13
  constraint horizontal L14
  constraint vertical L15
  constraint horizontal L16
  constraint vertical L17
  constraint horizontal L18
  constraint vertical L19
  constraint horizontal L31
  constraint vertical L30
  constraint horizontal L28
  constraint vertical L29
  constraint horizontal L35
  constraint vertical L34
  constraint horizontal L32
  constraint vertical L33
  constraint horizontal L27
  constraint vertical L26
  constraint horizontal L24
  constraint vertical L25
  constraint horizontal L23
  constraint vertical L20
  constraint horizontal L21
  constraint vertical L22
  constraint horizontal L46
  constraint vertical L44
  constraint horizontal L45
  constraint vertical L47
  constraint horizontal L40
  constraint vertical L41
  constraint horizontal L43
  constraint vertical L42
  constraint horizontal L48
  constraint vertical L49
  constraint horizontal L51
  constraint vertical L50
  constraint horizontal L39
  constraint vertical L36
  constraint horizontal L37
  constraint vertical L38
  measures "d194" distance of L12.start L12.end
  measures "d195" distance of L12.start L14.end
  measures "d198" distance of L16.start L16.end
  measures "d199" distance of L16.start L18.end
  measures "d200" distance of L26.start L25.end
  measures "d201" distance of L25.end L24.end
  measures "d202" distance of L22.end L20.start
  measures "d203" distance of L22.end L21.end
  measures "d204" distance of L48.start L48.end
  measures "d205" distance of L48.start L50.start
  measures "d206" distance of L38.end L36.start
  measures "d207" distance of L38.end L37.end
extrude "Extrude26" add sketch "Sketch24" along normal blind 9 contours L4 L5 L7 L12 L13 L15 L18 | L7 L8 L15 L18 | L5 L8 L13 L18 | L8 L9 L10 L15 L16 L18 L19 | L8 L10 L11 L13 L16 L17 L18 | L7 L10 L15 L16 | L5 L10 L13 L16 | L5 L6 L7 L13 L14 L15 L16 | L20 L21 L23 L26 L32 L33 L35 | L23 L26 L30 L32 | L23 L24 L25 L26 L28 L29 L30 | L21 L25 L26 L27 L29 L30 L31 | L21 L26 L30 L35 | L23 L25 L29 L32 | L21 L25 L29 L35 | L21 L22 L23 L25 L32 L34 L35 | L36 L37 L39 L40 L42 L43 L49 | L39 L43 L44 L49 | L39 L44 L45 L47 L49 L50 L51 | L37 L44 L46 L47 L48 L49 L50 | L37 L40 L44 L49 | L39 L43 L47 L50 | L37 L40 L47 L50 | L37 L38 L39 L40 L41 L43 L50 bodies 6
fillet "Fillet7" radius 1 8 edges at (45.25, 16, 10) (26, 17, 5) (27, 9, 10) (26, 1, 5) (45.25, 2, 10) (64.5, 17, 5) (63.5, 9, 10) (64.5, 1, 5) on bodies 6
move_body "Move11" bodies 6 to x (1, 0, 0) y (0, 1, 0) z (0, 0, 1) at (-45.2529, -8.3242, 12.2176)
sketch "Sketch25" plane through (0, 0, 0) normal (0, 0, 1) x (1, 0, 0)
  line L0 (30, 0) -> (79.5, 0)
  line L1 (79.5, 0) -> (79.5, 18)
  line L2 (79.5, 18) -> (30, 18)
  line L3 (30, 18) -> (30, 0)
  dimension "d212" = 49.5
  dimension "d213" = 18
  constraint horizontal L0
  constraint vertical L1
  constraint horizontal L2
  constraint vertical L3
  measures "d212" distance of L0.start L0.end
  measures "d213" distance of L0.start L2.end
extrude "Extrude27" add sketch "Sketch25" along normal blind 10 separate body makes body 7
sketch "Sketch26" plane through (0, 0, 0) normal (0, -1, 0) x (1, 0, 0)
  line L0 (30, 0) -> (79.5, 0)
  line L1 (79.5, 0) -> (79.5, 10)
  line L2 (79.5, 10) -> (30, 10)
  line L3 (30, 10) -> (30, 0)
  line L4 (30, 10) -> (32, 10)
  line L5 (32, 10) -> (30, 0)
  line L6 (30, 0) -> (30, 10)
  line L7 (79.5, 10) -> (77.5, 10)
  line L8 (77.5, 10) -> (79.5, 0)
  line L9 (79.5, 0) -> (79.5, 10)
  dimension "d216" = 2
  constraint coincident L2.end L3.start
  constraint coincident L2 L4.end
  constraint coincident L0.start L3.end
  constraint coincident L1.end L2.start
  constraint perpendicular L1 L7
  constraint coincident L0.end L1.start
  measures "d216" distance of L1.end L7.end
sketch "Sketch27" plane through (79.5, 0, 0) normal (1, 0, 0) x (0, 0, -1)
  line L0 (0, 0) -> (0, 18)
  line L1 (0, 18) -> (-10, 18)
  line L2 (-10, 18) -> (-10, 0)
  line L3 (-10, 0) -> (0, 0)
  line L4 (-10, 0) -> (-10, 2)
  line L5 (-10, 2) -> (0, 0)
  line L6 (0, 0) -> (-10, 0)
  line L7 (-10, 18) -> (-10, 16)
  line L8 (-10, 16) -> (0, 18)
  line L9 (0, 18) -> (-10, 18)
  constraint coincident L2.end L3.start
  constraint coincident L2 L4.end
  constraint coincident L0.start L3.end
  constraint coincident L1.end L2.start
  constraint coincident L2 L7.end
  constraint coincident L0.end L1.start
extrude "Extrude28" cut sketch "Sketch27" against normal blind 55 contours L2 L3 L4 L5 L6 | L1 L2 L7 L8 L9 bodies 7
extrude "Extrude29" cut sketch "Sketch26" against normal blind 21 contours L2 L3 L4 L5 L6 | L1 L2 L7 L8 L9 bodies 7
shell "Shell8" thickness 1 removed faces 1 at (46.5, 12, 0) on bodies 7
sketch "Sketch28" plane through (0, 0, 9) normal (0, 0, -1) x (-1, 0, 0)
  line L0 (-76.6802, 15.1802) -> (-76.6802, 2.8198)
  line L1 (-76.6802, 2.8198) -> (-32.8198, 2.8198)
  line L2 (-32.8198, 2.8198) -> (-32.8198, 15.1802)
  line L3 (-32.8198, 15.1802) -> (-76.6802, 15.1802)
  line L4 (-54.2, 11) -> (-55.3, 11)
  line L5 (-55.3, 11) -> (-55.3, 7)
  line L6 (-55.3, 7) -> (-54.2, 7)
  line L7 (-54.2, 7) -> (-54.2, 11)
  line L8 (-52.75, 8.375) -> (-56.75, 8.375)
  line L9 (-56.75, 8.375) -> (-56.75, 9.625)
  line L10 (-56.75, 9.625) -> (-52.75, 9.625)
  line L11 (-52.75, 9.625) -> (-52.75, 8.375)
  line L12 (-56.3, 6) -> (-53.2, 6)
  line L13 (-53.2, 6) -> (-53.2, 12)
  line L14 (-53.2, 12) -> (-56.3, 12)
  line L15 (-56.3, 12) -> (-56.3, 6)
  line L16 (-57.75, 10.625) -> (-51.75, 10.625)
  line L17 (-51.75, 10.625) -> (-51.75, 7.375)
  line L18 (-51.75, 7.375) -> (-57.75, 7.375)
  line L19 (-57.75, 7.375) -> (-57.75, 10.625)
  line L20 (-52.75, 8.375) -> (-56.75, 8.375)
  line L21 (-56.75, 8.375) -> (-56.75, 9.625)
  line L22 (-56.75, 9.625) -> (-52.75, 9.625)
  line L23 (-52.75, 9.625) -> (-52.75, 8.375)
  line L24 (-51.75, 7.375) -> (-57.75, 7.375)
  line L25 (-57.75, 7.375) -> (-57.75, 10.625)
  line L26 (-51.75, 10.625) -> (-51.75, 7.375)
  line L27 (-57.75, 10.625) -> (-51.75, 10.625)
  line L28 (-54.2, 7) -> (-54.2, 11)
  line L29 (-54.2, 11) -> (-55.3, 11)
  line L30 (-55.3, 7) -> (-54.2, 7)
  line L31 (-55.3, 11) -> (-55.3, 7)
  line L32 (-53.2, 12) -> (-56.3, 12)
  line L33 (-56.3, 12) -> (-56.3, 6)
  line L34 (-53.2, 6) -> (-53.2, 12)
  line L35 (-56.3, 6) -> (-53.2, 6)
  line L36 (-52.75, 8.375) -> (-56.75, 8.375)
  line L37 (-56.75, 8.375) -> (-56.75, 9.625)
  line L38 (-56.75, 9.625) -> (-52.75, 9.625)
  line L39 (-52.75, 9.625) -> (-52.75, 8.375)
  line L40 (-51.75, 7.375) -> (-57.75, 7.375)
  line L41 (-57.75, 7.375) -> (-57.75, 10.625)
  line L42 (-51.75, 10.625) -> (-51.75, 7.375)
  line L43 (-57.75, 10.625) -> (-51.75, 10.625)
  line L44 (-54.2, 7) -> (-54.2, 11)
  line L45 (-54.2, 11) -> (-55.3, 11)
  line L46 (-55.3, 7) -> (-54.2, 7)
  line L47 (-55.3, 11) -> (-55.3, 7)
  line L48 (-53.2, 12) -> (-56.3, 12)
  line L49 (-56.3, 12) -> (-56.3, 6)
  line L50 (-53.2, 6) -> (-53.2, 12)
  line L51 (-56.3, 6) -> (-53.2, 6)
  line L52 (-40.675, 8.375) -> (-44.675, 8.375)
  line L53 (-44.675, 8.375) -> (-44.675, 9.625)
  line L54 (-44.675, 9.625) -> (-40.675, 9.625)
  line L55 (-40.675, 9.625) -> (-40.675, 8.375)
  line L56 (-39.675, 7.375) -> (-45.675, 7.375)
  line L57 (-45.675, 7.375) -> (-45.675, 10.625)
  line L58 (-39.675, 10.625) -> (-39.675, 7.375)
  line L59 (-45.675, 10.625) -> (-39.675, 10.625)
  line L60 (-42.125, 7) -> (-42.125, 11)
  line L61 (-42.125, 11) -> (-43.225, 11)
  line L62 (-43.225, 7) -> (-42.125, 7)
  line L63 (-43.225, 11) -> (-43.225, 7)
  line L64 (-41.125, 12) -> (-44.225, 12)
  line L65 (-44.225, 12) -> (-44.225, 6)
  line L66 (-41.125, 6) -> (-41.125, 12)
  line L67 (-44.225, 6) -> (-41.125, 6)
  line L68 (-64.825, 8.375) -> (-68.825, 8.375)
  line L69 (-68.825, 8.375) -> (-68.825, 9.625)
  line L70 (-68.825, 9.625) -> (-64.825, 9.625)
  line L71 (-64.825, 9.625) -> (-64.825, 8.375)
  line L72 (-63.825, 7.375) -> (-69.825, 7.375)
  line L73 (-69.825, 7.375) -> (-69.825, 10.625)
  line L74 (-63.825, 10.625) -> (-63.825, 7.375)
  line L75 (-69.825, 10.625) -> (-63.825, 10.625)
  line L76 (-66.275, 7) -> (-66.275, 11)
  line L77 (-66.275, 11) -> (-67.375, 11)
  line L78 (-67.375, 7) -> (-66.275, 7)
  line L79 (-67.375, 11) -> (-67.375, 7)
  line L80 (-65.275, 12) -> (-68.375, 12)
  line L81 (-68.375, 12) -> (-68.375, 6)
  line L82 (-65.275, 6) -> (-65.275, 12)
  line L83 (-68.375, 6) -> (-65.275, 6)
  dimension "d231" = 3.1
  dimension "d232" = 6
  dimension "d235" = 6
  dimension "d236" = 3.25
  dimension "d237" = 3.1
  dimension "d238" = 6
  dimension "d239" = 6
  dimension "d240" = 3.25
  dimension "d241" = 3.1
  dimension "d242" = 6
  dimension "d243" = 6
  dimension "d244" = 3.25
  dimension "d245" = 3.1
  dimension "d246" = 6
  dimension "d247" = 6
  dimension "d248" = 3.25
  dimension "d249" = 3.1
  dimension "d250" = 6
  dimension "d251" = 6
  dimension "d252" = 3.25
  constraint horizontal L4
  constraint vertical L5
  constraint horizontal L6
  constraint vertical L7
  constraint horizontal L8
  constraint vertical L9
  constraint horizontal L10
  constraint vertical L11
  constraint horizontal L12
  constraint vertical L13
  constraint horizontal L14
  constraint vertical L15
  constraint horizontal L16
  constraint vertical L17
  constraint horizontal L18
  constraint vertical L19
  constraint horizontal L29
  constraint vertical L31
  constraint horizontal L30
  constraint vertical L28
  constraint horizontal L20
  constraint vertical L21
  constraint horizontal L22
  constraint vertical L23
  constraint horizontal L35
  constraint vertical L34
  constraint horizontal L32
  constraint vertical L33
  constraint horizontal L27
  constraint vertical L26
  constraint horizontal L24
  constraint vertical L25
  constraint horizontal L45
  constraint vertical L47
  constraint horizontal L46
  constraint vertical L44
  constraint horizontal L36
  constraint vertical L37
  constraint horizontal L38
  constraint vertical L39
  constraint horizontal L51
  constraint vertical L50
  constraint horizontal L48
  constraint vertical L49
  constraint horizontal L43
  constraint vertical L42
  constraint horizontal L40
  constraint vertical L41
  constraint horizontal L61
  constraint vertical L63
  constraint horizontal L62
  constraint vertical L60
  constraint horizontal L52
  constraint vertical L53
  constraint horizontal L54
  constraint vertical L55
  constraint horizontal L67
  constraint vertical L66
  constraint horizontal L64
  constraint vertical L65
  constraint horizontal L59
  constraint vertical L58
  constraint horizontal L56
  constraint vertical L57
  constraint horizontal L77
  constraint vertical L79
  constraint horizontal L78
  constraint vertical L76
  constraint horizontal L68
  constraint vertical L69
  constraint horizontal L70
  constraint vertical L71
  constraint horizontal L83
  constraint vertical L82
  constraint horizontal L80
  constraint vertical L81
  constraint horizontal L75
  constraint vertical L74
  constraint horizontal L72
  constraint vertical L73
  measures "d231" distance of L12.start L12.end
  measures "d232" distance of L12.start L14.end
  measures "d235" distance of L16.start L16.end
  measures "d236" distance of L16.start L18.end
  measures "d237" distance of L12.end L12.start
  measures "d238" distance of L14.end L12.start
  measures "d239" distance of L16.end L16.start
  measures "d240" distance of L18.end L16.start
  measures "d241" distance of L12.end L12.start
  measures "d242" distance of L14.end L12.start
  measures "d243" distance of L16.end L16.start
  measures "d244" distance of L18.end L16.start
  measures "d245" distance of L66.start L65.end
  measures "d246" distance of L64.end L65.end
  measures "d247" distance of L58.start L57.end
  measures "d248" distance of L56.end L57.end
  measures "d249" distance of L82.start L81.end
  measures "d250" distance of L80.end L81.end
  measures "d251" distance of L74.start L73.end
  measures "d252" distance of L72.end L73.end
extrude "Extrude30" add sketch "Sketch28" along normal blind 9 contours L4 L5 L7 L13 L14 L15 L16 L27 L28 L29 L31 L32 L33 L34 L43 L44 L45 L47 L48 L49 L50 | L7 L10 L13 L16 L22 L27 L28 L34 L38 L43 L44 L50 | L5 L10 L15 L16 L22 L27 L31 L33 L38 L43 L47 L49 | L8 L10 L11 L13 L16 L17 L18 L20 L22 L23 L24 L26 L27 L34 L36 L38 L39 L40 L42 L43 L50 | L8 L9 L10 L15 L16 L18 L19 L20 L21 L22 L24 L25 L27 L33 L36 L37 L38 L40 L41 L43 L49 | L7 L8 L13 L18 L20 L24 L28 L34 L36 L40 L44 L50 | L5 L8 L15 L18 L20 L24 L31 L33 L36 L40 L47 L49 | L5 L6 L7 L12 L13 L15 L18 L24 L28 L30 L31 L33 L34 L35 L40 L44 L46 L47 L49 L50 L51 | L52 L54 L55 L56 L58 L59 L66 | L52 L56 L60 L66 | L56 L60 L62 L63 L65 L66 L67 | L54 L59 L60 L66 | L52 L56 L63 L65 | L59 L60 L61 L63 L64 L65 L66 | L52 L53 L54 L56 L57 L59 L65 | L54 L59 L63 L65 | L68 L70 L71 L72 L74 L75 L82 | L68 L72 L76 L82 | L72 L76 L78 L79 L81 L82 L83 | L70 L75 L76 L82 | L68 L72 L79 L81 | L75 L76 L77 L79 L80 L81 L82 | L68 L69 L70 L72 L73 L75 L81 | L70 L75 L79 L81 bodies 7
fillet "Fillet8" radius 1 8 edges at (54.75, 16, 10) (32, 9, 10) (54.75, 2, 10) (31, 17, 5) (31, 1, 5) (77.5, 9, 10) (78.5, 17, 5) (78.5, 1, 5) on bodies 7
move_body "Move12" bodies 7 to x (1, 0, 0) y (0, 1, 0) z (0, 0, 1) at (-54.7471, -8.3198, 12.2152)
sketch "Sketch29" plane through (0, 0, 0) normal (0, 0, 1) x (1, 0, 0)
  line L0 (40, 0) -> (71.5, 0)
  line L1 (71.5, 0) -> (71.5, 18)
  line L2 (71.5, 18) -> (40, 18)
  line L3 (40, 18) -> (40, 0)
  dimension "d257" = 31.5
  dimension "d258" = 18
  constraint horizontal L0
  constraint vertical L1
  constraint horizontal L2
  constraint vertical L3
  measures "d257" distance of L0.start L0.end
  measures "d258" distance of L0.start L2.end
extrude "Extrude31" add sketch "Sketch29" along normal blind 10 separate body makes body 8